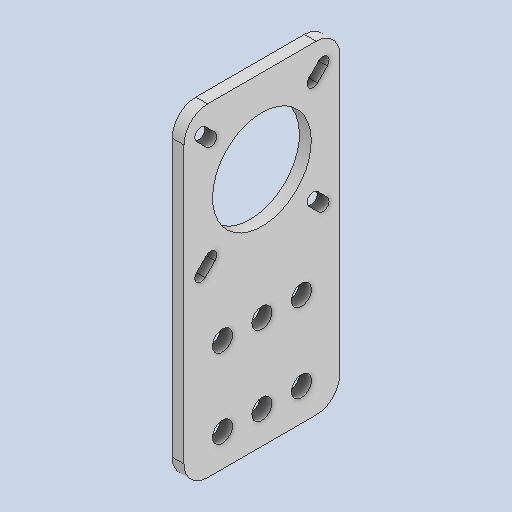
# Autodesk Inventor part: HCMUTE-CDT23-OP_GA-STEP-42
Saved by Autodesk Inventor 2023 (Build 270158000, 158)
## iProperties
Created: 2023-11-14
Part Number: HCMUTE-CDT23-OP_GA-STEP-42
Material: Generic
Document SubType Name: Sheet Metal
Designer: havie
Density: 1 g/cm^3
Sheet Metal Rule: Default_mm
Appearance: Default
Author: havie
Autodesk Inventor part; units mm, degrees
ref_plane "YZ Plane" through (0, 0, 0) normal (1, 0, 0) x (0, 1, 0)
ref_plane "XZ Plane" through (0, 0, 0) normal (0, 1, 0) x (-1, 0, 0)
ref_plane "XY Plane" through (0, 0, 0) normal (0, 0, 1) x (1, 0, 0)
sketch "Sketch1" plane through (0, 0, 0) normal (1, 0, 0) x (0, 1, 0)
  line L0 (41, 19.75) -> (-41, 19.75)
  line L1 (-41, 19.75) -> (-41, -19.75)
  line L2 (-41, -19.75) -> (41, -19.75)
  line L3 (41, -19.75) -> (41, 19.75)
  line L4 (41, 19.75) -> (-41, -19.75) construction
  line L5 (-41, 19.75) -> (41, -19.75) construction
  circle A0 centre (19.75, 0) radius 12.5
  line L6 (35.2464, 15.4749) -> (32.7715, 13) construction
  line L7 (34.1504, 16.5709) -> (31.6755, 14.096)
  line L8 (33.8675, 11.904) -> (36.3424, 14.3789)
  arc A1 (36.3424, 14.3789) -> (34.1504, 16.5709) centre (35.2464, 15.4749) ccw
  arc A2 (31.6755, 14.096) -> (33.8675, 11.904) centre (32.7715, 13) ccw
  line L9 (35.2464, -15.4749) -> (32.7715, -13) construction
  line L10 (36.3424, -14.3789) -> (33.8675, -11.904)
  line L11 (31.6755, -14.096) -> (34.1504, -16.5709)
  arc A3 (34.1504, -16.5709) -> (36.3424, -14.3789) centre (35.2464, -15.4749) ccw
  arc A4 (33.8675, -11.904) -> (31.6755, -14.096) centre (32.7715, -13) ccw
  line L12 (6.7715, -13) -> (4.2966, -15.4749) construction
  line L13 (5.6755, -11.904) -> (3.2006, -14.3789)
  line L14 (5.3927, -16.5709) -> (7.8675, -14.096)
  arc A5 (7.8675, -14.096) -> (5.6755, -11.904) centre (6.7715, -13) ccw
  arc A6 (3.2006, -14.3789) -> (5.3927, -16.5709) centre (4.2966, -15.4749) ccw
  line L15 (6.7715, 13) -> (4.2966, 15.4749) construction
  line L16 (7.8675, 14.096) -> (5.3927, 16.5709)
  line L17 (3.2006, 14.3789) -> (5.6755, 11.904)
  arc A7 (5.6755, 11.904) -> (7.8675, 14.096) centre (6.7715, 13) ccw
  arc A8 (5.3927, 16.5709) -> (3.2006, 14.3789) centre (4.2966, 15.4749) ccw
  line L18 (-57.4, 0) -> (57.4, 0) construction
  line L19 (0, -27.65) -> (0, 27.65) construction
  circle A9 centre (-32.8, 10) radius 2.55
  circle A10 centre (-32.8, 0) radius 2.55
  circle A11 centre (-32.8, -10) radius 2.55
  circle A12 centre (-12.8, 10) radius 2.55
  circle A13 centre (-12.8, -10) radius 2.55
  circle A14 centre (-12.8, 0) radius 2.55
  point P0 (0, 0)
  point P1 (34.009, 14.2374)
  point P2 (34.009, -14.2374)
  point P3 (5.5341, -14.2374)
  point P4 (5.5341, 14.2374)
  dimension "d0" = 82
  dimension "d1" = 39.5
  dimension "d2" = 25
  dimension "d3" = 21.25
  dimension "d4" = 45
  dimension "d5" = 45
  dimension "d6" = 45
  dimension "d7" = 3.5
  dimension "d8" = 3.5
  dimension "d9" = 3.5
  dimension "d10" = 3.5
  dimension "d11" = 3.1
  dimension "d12" = 3.1
  dimension "d13" = 3.1
  dimension "d14" = 3.1
  dimension "d16" = 18.4
  dimension "d17" = 26
  dimension "d19" = 26
  dimension "d20" = 13
  dimension "d21" = 5.1
  dimension "d22" = 5.1
  dimension "d23" = 5.1
  dimension "d24" = 5.1
  dimension "d25" = 5.1
  dimension "d26" = 5.1
  dimension "d27" = 8.2
  dimension "d28" = 9.75
  dimension "d29" = 9.75
  dimension "d30" = 20
  measures "d0" distance of L1.end L2.end
  measures "d1" distance of L0.end L1.end
  measures "d2" diameter of A0
  measures "d3" distance from line of L3 A0.centre
  measures "d4" angle of L19 L15
  measures "d5" angle of L18 L6
  measures "d6" angle of L18 L9
  measures "d7" distance of L8.start L8.end
  measures "d8" distance of L10.start L10.end
  measures "d9" distance of L14.start L14.end
  measures "d10" distance of L16.start L16.end
  measures "d11" distance between parallel lines of L16 L17
  measures "d12" distance between parallel lines of L13 L14
  measures "d13" distance between parallel lines of L11 L10
  measures "d14" distance between parallel lines of L7 L8
  measures "d16" distance of A0.centre L6.end
  measures "d17" distance of L6.end L15.start
  measures "d19" distance of L9.end L6.end
  measures "d20" distance from line of L18 L6.end
  measures "d21" diameter of A9
  measures "d22" diameter of A12
  measures "d23" diameter of A14
  measures "d24" diameter of A13
  measures "d25" diameter of A11
  measures "d26" diameter of A10
  measures "d27" distance from line of L1 A9.centre
  measures "d28" distance from line of L0 A12.centre
  measures "d29" distance from line of L2 A13.centre
  measures "d30" distance of A14.centre A10.centre
extrude "Plate1" add sketch "Sketch1" along normal mid plane 3
fillet "Corner Round1" radius 6 4 edges at (0, 41, 19.75) (0, 41, -19.75) (0, -41, 19.75) (0, -41, -19.75)
equation "\"d8\" = d7"
equation "\"d22\" = d21"
equation "\"d23\" = d22"
equation "\"d24\" = d23"
equation "\"d25\" = d24"
equation "\"d26\" = d24"
equation "\"d31\" = Thickness"
equation "\"BendRadius\" = Thickness"
equation "\"BendReliefWidth\" = Thickness"
equation "\"BendReliefDepth\" = 0.5 * Thickness"
equation "\"CornerReliefSize\" = 4 * Thickness"
equation "\"MinimumRemnant\" = 2 * Thickness"
equation "\"TransitionRadius\" = BendRadius"
equation "\"JacobiRadiusSize\" = BendRadius"
equation "\"GapSize\" = Thickness"
equation "\"Thickness\" = 3"
body "Solid1"
